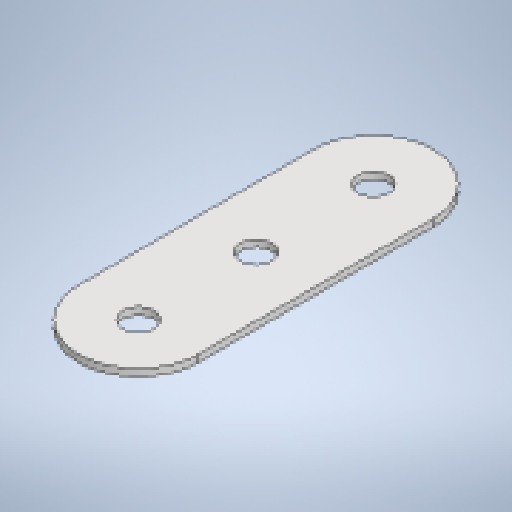
# Autodesk Inventor part: IntakeHolder1.2
Saved by Autodesk Inventor 2023 (Build 270158000, 158)
## iProperties
Created: 2022-09-18
Part Number: IntakeHolder1.2
Material: Generic
Document SubType Name: Modeling
Designer: deli
Density: 1 g/cm^3
Appearance: Default
Author: deli
Autodesk Inventor part; units mm, degrees
ref_plane "YZ Plane" through (0, 0, 0) normal (1, 0, 0) x (0, 1, 0)
ref_plane "XZ Plane" through (0, 0, 0) normal (0, 1, 0) x (-1, 0, 0)
ref_plane "XY Plane" through (0, 0, 0) normal (0, 0, 1) x (1, 0, 0)
sketch "Sketch1" plane through (0, 0, 0) normal (0, 1, 0) x (-1, 0, 0)
  arc A0 (-83.3096, 40.016) -> (-29.7548, 40.016) centre (-56.5322, 40.016) ccw
  circle A1 centre (-56.5322, 40.016) radius 7
  circle A2 centre (-56.5322, 92.516) radius 7
  circle A3 centre (-56.5322, 40.016) radius 25.4 construction
  circle A4 centre (-56.5322, 92.516) radius 25.4 construction
  line L0 (-29.7548, 145.016) -> (-29.7548, 40.016)
  line L1 (-83.3096, 145.016) -> (-83.3096, 40.016)
  circle A5 centre (14.2452, 64.2849) radius 50.8 construction
  arc A6 (58.2452, 40.016) -> (111.8, 40.016) centre (85.0226, 40.016) ccw
  circle A7 centre (85.0226, 40.016) radius 7
  circle A8 centre (85.0226, 92.516) radius 7
  circle A9 centre (85.0226, 40.016) radius 25.4 construction
  circle A10 centre (85.0226, 92.516) radius 25.4 construction
  line L2 (58.2452, 81.4638) -> (58.2452, 40.016)
  line L3 (111.8, 120.0259) -> (111.8, 40.016)
  line L4 (-56.5322, 92.516) -> (-56.5322, 40.016) construction
  line L5 (-36.3164, 59.3687) -> (-28.6945, 37.1404) construction
  line L6 (-31.1322, 40.0031) -> (-36.4845, 55.6125) construction
  line L7 (-56.5322, 40.016) -> (14.2452, 64.2849) construction
  circle A11 centre (-56.5322, 145.016) radius 7
  arc A12 (-29.7548, 145.016) -> (-83.3096, 145.016) centre (-56.5322, 145.016) ccw
  circle A13 centre (14.2452, 11.7849) radius 50.8 construction
  point P0 (0, 0)
  dimension "d2" = 14
  dimension "d3" = 14
  dimension "d4" = 50.8
  dimension "d5" = 50.8
  dimension "d11" = 101.6
  dimension "d12" = 1.3774
  dimension "d13" = 14
  dimension "d14" = 14
  dimension "d16" = 1.3774
  dimension "d17" = 1.3774
  dimension "d18" = 50.8
  dimension "d19" = 50.8
  dimension "d24" = 52.5
  dimension "d25" = 52.5
  dimension "d28" = 1.3774
  dimension "d30" = 88
  dimension "d33" = 0
  dimension "d34" = 1.3774
  dimension "d35" = 14
  dimension "d36" = 52.5
  dimension "d39" = 101.6
  constraints: 16 end point, 14 centre point, 12 tangent, 10 point on circle, 6 coincident, 3 parallel, 2 concentric, 1 perpendicular, 1 vertical
  measures "d2" diameter of A1
  measures "d3" diameter of A2
  measures "d4" diameter of A3
  measures "d5" diameter of A4
  measures "d11" diameter of A5
  measures "d12" distance edge to line of A9 L2
  measures "d13" diameter of A7
  measures "d14" diameter of A8
  measures "d16" distance edge to line of A3 L0
  measures "d17" distance edge to line of A4 L0
  measures "d18" diameter of A10
  measures "d19" diameter of A9
  measures "d24" distance of A1.centre A2.centre
  measures "d25" distance of A7.centre A8.centre
  measures "d28" distance edge to line of A10 L2
  measures "d30" distance between parallel lines of L0 L2
  measures "d33" vertical distance of A2.centre A10.centre
  measures "d34" distance between parallel lines of L6 L5
  measures "d35" diameter of A11
  measures "d36" distance of A2.centre A11.centre
  measures "d39" diameter of A13
extrude "Extrusion1" add sketch "Sketch1" along normal blind 3.175 contours L1 A12 L0 A0
equation "\"d2\" = d0"
equation "\"d3\" = d0"
equation "\"d5\" = d4"
equation "\"d12\" = d16"
equation "\"d13\" = d0"
equation "\"d14\" = d0"
equation "\"d17\" = d16"
equation "\"d18\" = d4"
equation "\"d19\" = d4"
equation "\"d25\" = d24"
equation "\"d28\" = d16"
equation "\"d10\" = d8"
equation "\"d0\" = 14"
equation "\"d8\" = 2"
body "Solid1"
